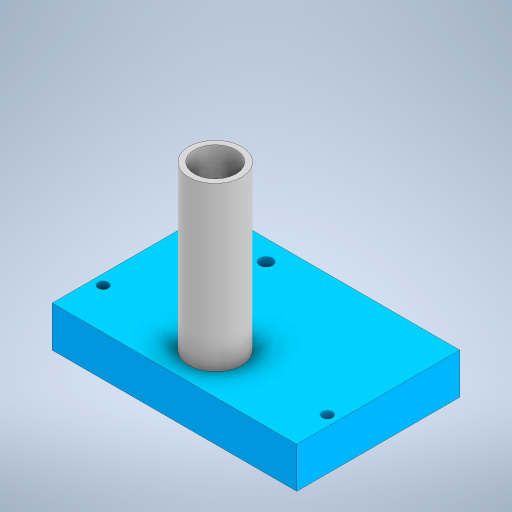
# Autodesk Inventor part: Bottom Plate For Side to Side Motion
Saved by Autodesk Inventor 2023.1 (Build 271208000, 208)
## iProperties
Created: 2022-12-21
Part Number: Bottom Plate For Side to Side Motion
Material: Generic
Document SubType Name: Modeling
Designer: shubh
Density: 1 g/cm^3
Appearance: Default
Author: shubh
Autodesk Inventor part; units mm, degrees
ref_plane "YZ Plane" through (0, 0, 0) normal (1, 0, 0) x (0, 1, 0)
ref_plane "XZ Plane" through (0, 0, 0) normal (0, 1, 0) x (-1, 0, 0)
ref_plane "XY Plane" through (0, 0, 0) normal (0, 0, 1) x (1, 0, 0)
sketch "Sketch1" plane through (0, 0, 0) normal (0, 1, 0) x (-1, 0, 0)
  line L0 (69.85, 63.5) -> (-82.55, 63.5)
  line L1 (-82.55, 63.5) -> (-82.55, -38.1)
  line L2 (-82.55, -38.1) -> (69.85, -38.1)
  line L3 (69.85, -38.1) -> (69.85, 63.5)
  circle A0 centre (25.4, -25.4) radius 3.9751
  circle A1 centre (63.5, 38.1) radius 3.175
  circle A2 centre (-76.2, 38.1) radius 3.175
  point P0 (0, 0)
  dimension "d0" = 101.6
  dimension "d1" = 152.4
  dimension "d3" = 38.1
  dimension "d4" = 7.9502
  dimension "d16" = 6.35
  dimension "d17" = 6.35
  dimension "d18" = 25.4
  dimension "d20" = 6.35
  dimension "d21" = 6.35
  dimension "d22" = 44.45
  dimension "d24" = 25.4
  dimension "d26" = 25.4
  constraints: 8 end point, 3 centre point, 2 parallel, 1 horizontal, 1 perpendicular
  measures "d0" distance of L2.end L0.start
  measures "d1" distance of L1.end L2.end
  measures "d3" distance from line of L2 point (0, 0)
  measures "d4" diameter of A0
  measures "d16" diameter of A1
  measures "d17" distance from line of L3 A1.centre
  measures "d18" distance from line of A1.centre L0
  measures "d20" diameter of A2
  measures "d21" distance from line of L1 A2.centre
  measures "d22" distance from line of L3 A0.centre
  measures "d24" horizontal distance of point (0, 0) A0.centre
  measures "d26" distance from line of L0 A2.centre
extrude "Extrusion1" add sketch "Sketch1" along normal blind 25.4
sketch "Sketch2" plane through (0, 25.4, 0) normal (0, 1, 0) x (1, 0, 0)
  circle A0 centre (6.35, -38.1) radius 16.51
  circle A1 centre (76.2, -38.1) radius 3.175 projected
  line L0 (82.55, -63.5) -> (82.55, 38.1) projected
  point P0 (0, 0)
  dimension "d7" = 33.02
  dimension "d25" = 76.2
  constraints: 1 centre point
  measures "d7" diameter of A0
  measures "d25" distance from line of L0 A0.centre
extrude "Extrusion2" add sketch "Sketch2" along normal blind 101.6 contours A0
sketch "Sketch3" plane through (6.35, 127, 38.1) normal (0, 1, 0) x (1, 0, 0)
  circle A0 centre (0, 0) radius 13.0175
  point P0 (-6.35, 38.1)
  dimension "d10" = 26.035
  constraints: 1 centre point
  measures "d10" diameter of A0
extrude "Extrusion3" cut sketch "Sketch3" against normal blind 41.91
sketch "Sketch4" plane through (6.35, 85.09, 38.1) normal (0, 1, 0) x (1, 0, 0)
  circle A0 centre (0, 0) radius 16.51 projected
  circle A1 centre (0, 0) radius 16.002
  point P0 (-6.35, 38.1)
  dimension "d13" = 32.004
  constraints: 1 centre point, 1 coincident
  measures "d13" diameter of A1
extrude "Extrusion4" cut sketch "Sketch4" against normal blind 59.69 contours A1
body "Solid1"
